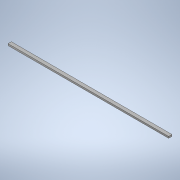
# Autodesk Inventor part: HFS5-4040-120
Saved by Autodesk Inventor 2020 (Build 240168000, 168)
## iProperties
Created: 2019-06-28
Part Number: HFS5-4040-120
Material: EN AC-51400-T5 Equiv.
Document SubType Name: Modeling
Designer: Mike
Density: 2.7 g/cm^3
Appearance: Generisch
Mass: 4147.2 g
Surface Area: 2320 cm^2
Volume: 1536 cm^3
Author: Mike
Autodesk Inventor part; units mm, degrees
ref_plane "YZ Plane" through (0, 0, 0) normal (1, 0, 0) x (0, 1, 0)
ref_plane "XZ Plane" through (0, 0, 0) normal (0, 1, 0) x (-1, 0, 0)
ref_plane "XY Plane" through (0, 0, 0) normal (0, 0, 1) x (1, 0, 0)
sketch "Skizze2" plane through (0, 0, 0) normal (1, 0, 0) x (0, 1, 0)
  line L0 (-10, -20) -> (10, -20)
  line L1 (10, -20) -> (10, 20)
  line L2 (10, 20) -> (-10, 20)
  line L3 (-10, 20) -> (-10, -20)
  line L4 (-10, -20) -> (10, 20) construction
  line L5 (10, -20) -> (-10, 20) construction
  point P0 (0, 0)
  dimension "d4" = 20
  dimension "d5" = 40
  constraints: 12 end point, 2 midpoint, 2 parallel, 1 horizontal, 1 perpendicular
  measures "d4" distance of L2.end L1.end
  measures "d5" distance of L1.end L0.end
extrude "Extrusion2" add sketch "Skizze2" along normal blind 1920
